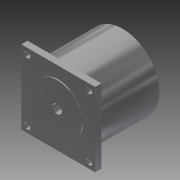
# Autodesk Inventor part: stepperMotorBody
Saved by Autodesk Inventor 2013 (Build 170138000, 138)
## iProperties
Created: 2013-02-24
Part Number: stepperMotorBody
Material: Steel, Galvanized
Document SubType Name: Modeling
Designer: Nano
Mass: 963.328 g
Surface Area: 165.043 cm^2
Volume: 122.717 cm^3
Density: 7.85 g/cm^3
Author: Nano
Autodesk Inventor part; units mm, degrees
ref_plane "YZ Plane" through (0, 0, 0) normal (1, 0, 0) x (0, 1, 0)
ref_plane "XZ Plane" through (0, 0, 0) normal (0, 1, 0) x (-1, 0, 0)
ref_plane "XY Plane" through (0, 0, 0) normal (0, 0, 1) x (1, 0, 0)
sketch "Sketch1" plane through (0, 0, 0) normal (0, 0, 1) x (1, 0, 0)
  line L0 (-28.1781, -28.1781) -> (28.1781, -28.1781)
  line L1 (28.1781, -28.1781) -> (28.1781, 28.1781)
  line L2 (28.1781, 28.1781) -> (-28.1781, 28.1781)
  line L3 (-28.1781, 28.1781) -> (-28.1781, -28.1781)
  line L4 (-28.1781, -28.1781) -> (28.1781, 28.1781) construction
  line L5 (28.1781, -28.1781) -> (-28.1781, 28.1781) construction
  circle A0 centre (-23.5732, 23.5732) radius 2.3813 projected
  circle A1 centre (23.5732, 23.5732) radius 2.3813 projected
  circle A2 centre (23.5732, -23.5732) radius 2.3813 projected
  circle A3 centre (-23.5732, -23.5732) radius 2.3813 projected
  circle A4 centre (0, 0) radius 3.556 projected
  dimension "d0" = 56.3563
  dimension "d1" = 56.3563
  constraints: 12 end point, 2 midpoint, 2 parallel, 1 perpendicular
  measures "d0" distance of L0.start L0.end
  measures "d1" distance of L1.end L0.end
extrude "Extrusion1" add sketch "Sketch1" against normal blind 4.7625
sketch "Sketch2" plane through (0, 0, 0) normal (0, 0, 1) x (1, 0, 0)
  circle A0 centre (0, 0) radius 3.556 projected
  circle A1 centre (0, 0) radius 3.556 projected
  circle A2 centre (0, 0) radius 19.05
  dimension "d4" = 38.1
  constraints: 1 centre point
  measures "d4" diameter of A2
extrude "Extrusion2" add sketch "Sketch2" along normal blind 0.7937
sketch "Sketch3" plane through (0, 0, -4.7625) normal (0, 0, -1) x (-1, 0, 0)
  circle A0 centre (0, 0) radius 3.556 projected
  circle A1 centre (0, 0) radius 27.94
  dimension "d7" = 55.88
  constraints: 1 centre point
  measures "d7" diameter of A1
extrude "Extrusion3" add sketch "Sketch3" along normal blind 44.45
body "Solid1"
